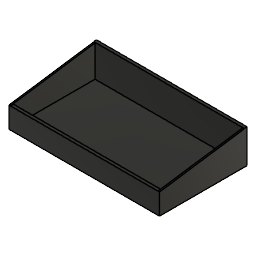
bin (Autodesk Fusion 360 design; units mm, degrees)
part number: 2026-08-18-18-57-01-469
Autodesk Fusion 360 part; units mm, degrees
sketch "Sketch1" plane through (0, 0, 0) normal (0, 0, 1) x (1, 0, 0)
  line L0 (0, 0) -> (201, 0)
  line L1 (201, 0) -> (201, 117)
  line L2 (201, 117) -> (0, 117)
  line L3 (0, 117) -> (0, 0)
extrude "Extrude1" add sketch "Sketch1" along normal blind 2.4 makes body 1
sketch "Sketch2" plane through (0, 0, 0) normal (0, 0, 1) x (1, 0, 0)
  line L0 (0, 0) -> (201, 0)
  line L1 (201, 0) -> (201, 4)
  line L2 (201, 4) -> (0, 4)
  line L3 (0, 4) -> (0, 0)
extrude "Extrude2" add sketch "Sketch2" along normal blind 28 separate body makes body 2
sketch "Sketch3" plane through (0, 0, 0) normal (0, 0, 1) x (1, 0, 0)
  line L0 (0, 113) -> (201, 113)
  line L1 (201, 113) -> (201, 117)
  line L2 (201, 117) -> (0, 117)
  line L3 (0, 117) -> (0, 113)
extrude "Extrude3" add sketch "Sketch3" along normal blind 45 separate body makes body 3
sketch "Sketch4" plane through (0, 0, 0) normal (1, 0, 0) x (0, 0, -1)
  line L0 (0, 0) -> (0, 117)
  line L1 (0, 117) -> (-45, 117)
  line L2 (-45, 117) -> (-28, 0)
  line L3 (-28, 0) -> (0, 0)
extrude "Extrude4" add sketch "Sketch4" along normal blind 2 separate body makes body 4
sketch "Sketch5" plane through (0, 0, 0) normal (1, 0, 0) x (0, 0, -1)
  line L0 (0, 0) -> (0, 117)
  line L1 (0, 117) -> (-45, 117)
  line L2 (-45, 117) -> (-28, 0)
  line L3 (-28, 0) -> (0, 0)
extrude "Extrude5" add sketch "Sketch5" along normal blind 2 from surface at 199 separate body makes body 5
combine "Combine1" operation add target body 1 tool bodies 2 3 4 5
named bodies: "Тело"
